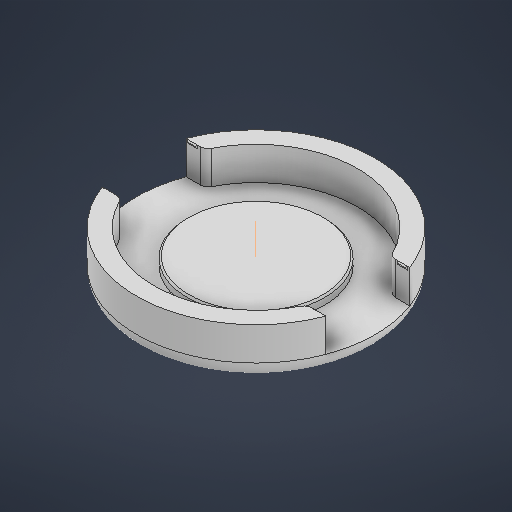
# Autodesk Inventor part: Head Plate Cover Cap
Saved by Autodesk Inventor 2026.1 (Build 301233000, 233)
## iProperties
Created: 2025-10-23
Part Number: Head Plate Cover Cap
Material: Generic
Document SubType Name: Modeling
Designer: mumin
Density: 1 g/cm^3
Appearance: Default
Author: mumin
Autodesk Inventor part; units mm, degrees
ref_plane "YZ Plane" through (0, 0, 0) normal (1, 0, 0) x (0, 1, 0)
ref_plane "XZ Plane" through (0, 0, 0) normal (0, 1, 0) x (-1, 0, 0)
ref_plane "XY Plane" through (0, 0, 0) normal (0, 0, 1) x (1, 0, 0)
sketch "Sketch1" plane through (0, 0, 0) normal (0, 1, 0) x (-1, 0, 0)
  circle A0 centre (0, 0) radius 42.1
  arc A1 (54.3341, 27.7273) -> (-54.3341, 27.7273) centre (0, 0) ccw
  line L0 (0, 0) -> (0, -61)
  line L1 (0, 0) -> (0, 0)
  line L2 (-117.5, 20) -> (-117.5, -20)
  line L3 (117.5, -20) -> (117.5, 20)
  line L4 (117.5, 25) -> (-117.5, -25) construction
  line L5 (-117.5, 25) -> (117.5, -25) construction
  line L6 (112.5, 25) -> (58.7878, 25)
  line L7 (-58.7878, 25) -> (-112.5, 25)
  line L8 (58.7878, -25) -> (112.5, -25)
  line L9 (-112.5, -25) -> (-58.7878, -25)
  arc A2 (-54.3341, -27.7273) -> (54.3341, -27.7273) centre (0, 0) ccw
  arc A3 (112.5, -25) -> (117.5, -20) centre (112.5, -20) ccw
  arc A4 (117.5, 20) -> (112.5, 25) centre (112.5, 20) ccw
  arc A5 (58.7878, -25) -> (54.3341, -27.7273) centre (58.7878, -30) ccw
  arc A6 (54.3341, 27.7273) -> (58.7878, 25) centre (58.7878, 30) ccw
  arc A7 (-54.3341, -27.7273) -> (-58.7878, -25) centre (-58.7878, -30) ccw
  arc A8 (-58.7878, 25) -> (-54.3341, 27.7273) centre (-58.7878, 30) ccw
  arc A9 (-117.5, -20) -> (-112.5, -25) centre (-112.5, -20) ccw
  arc A10 (-112.5, 25) -> (-117.5, 20) centre (-112.5, 20) ccw
  circle A11 centre (0, 0) radius 41.4
  circle A12 centre (0, 0) radius 67
  arc A13 (58.7878, -25.6) -> (54.8686, -28) centre (58.7878, -30) ccw
  line L10 (58.7878, -25.6) -> (112.5, -25.6)
  arc A14 (112.5, -25.6) -> (118.1, -20) centre (112.5, -20) ccw
  line L11 (118.1, -20) -> (118.1, 20)
  arc A15 (118.1, 20) -> (112.5, 25.6) centre (112.5, 20) ccw
  line L12 (112.5, 25.6) -> (58.7878, 25.6)
  arc A16 (54.8686, 28) -> (58.7878, 25.6) centre (58.7878, 30) ccw
  arc A17 (54.8686, 28) -> (-54.8686, 28) centre (0, 0) ccw
  arc A18 (-58.7878, 25.6) -> (-54.8686, 28) centre (-58.7878, 30) ccw
  line L13 (-58.7878, 25.6) -> (-112.5, 25.6)
  arc A19 (-112.5, 25.6) -> (-118.1, 20) centre (-112.5, 20) ccw
  line L14 (-118.1, 20) -> (-118.1, -20)
  arc A20 (-118.1, -20) -> (-112.5, -25.6) centre (-112.5, -20) ccw
  line L15 (-112.5, -25.6) -> (-58.7878, -25.6)
  arc A21 (-54.8686, -28) -> (-58.7878, -25.6) centre (-58.7878, -30) ccw
  arc A22 (-54.8686, -28) -> (54.8686, -28) centre (0, 0) ccw
  circle A23 centre (0, 0) radius 72
  line L16 (-112.5, 25.3) -> (-58.7878, 25.3)
  arc A24 (-58.7878, 25.3) -> (-54.6014, 27.8636) centre (-58.7878, 30) ccw
  arc A25 (54.6014, 27.8636) -> (-54.6014, 27.8636) centre (0, 0) ccw
  arc A26 (54.6014, 27.8636) -> (58.7878, 25.3) centre (58.7878, 30) ccw
  line L17 (58.7878, 25.3) -> (112.5, 25.3)
  arc A27 (117.8, 20) -> (112.5, 25.3) centre (112.5, 20) ccw
  line L18 (117.8, 20) -> (117.8, -20)
  arc A28 (112.5, -25.3) -> (117.8, -20) centre (112.5, -20) ccw
  line L19 (112.5, -25.3) -> (58.7878, -25.3)
  arc A29 (58.7878, -25.3) -> (54.6014, -27.8636) centre (58.7878, -30) ccw
  arc A30 (-54.6014, -27.8636) -> (54.6014, -27.8636) centre (0, 0) ccw
  arc A31 (-54.6014, -27.8636) -> (-58.7878, -25.3) centre (-58.7878, -30) ccw
  line L20 (-58.7878, -25.3) -> (-112.5, -25.3)
  arc A32 (-117.8, -20) -> (-112.5, -25.3) centre (-112.5, -20) ccw
  line L21 (-117.8, -20) -> (-117.8, 20)
  arc A33 (-112.5, 25.3) -> (-117.8, 20) centre (-112.5, 20) ccw
  point P0 (0, 0)
  point P1 (0, -61)
  point P2 (55.6417, -25)
  point P3 (55.6417, 25)
  point P4 (-55.6417, 25)
  point P5 (-55.6417, -25)
  point P6 (61.9164, 25.6)
  point P7 (-61.9164, 25.6)
  point P8 (-61.9164, -25.6)
  point P9 (61.9164, -25.6)
  point P10 (-67.2952, -25.6)
  point P11 (67.2952, -25.6)
  point P12 (67.2952, 25.6)
  point P13 (-67.2952, 25.6)
  point P14 (-67.4085, -25.3)
  point P15 (67.4085, -25.3)
  point P16 (-67.4085, 25.3)
  point P17 (67.4085, 25.3)
  dimension "d0" = 84.2
  dimension "d1" = 61
  dimension "d2" = 235
  dimension "d3" = 50
  dimension "d4" = 5
  dimension "d5" = 0.7
  dimension "d6" = 134
  dimension "d7" = 0.6
  dimension "d19" = 5
  dimension "d21" = 0.3
  constraints: 64 point on circle, 44 end point, 34 centre point, 16 tangent, 15 parallel, 12 point on line, 7 equal radius, 6 perpendicular, 5 coincident, 3 horizontal, 2 midpoint, 1 vertical, 1 vertical alignment, 30 other
  measures "d0" diameter of A0
  measures "d1" radius of A1
  measures "d2" distance of L5.end L4.end
  measures "d3" distance of L4.end L5.start
  measures "d4" radius of A3
  measures "d5" radial gap between concentric circles of A0 A11
  measures "d6" diameter of A12
  measures "d7" radial gap between concentric circles of A2 A22
  measures "d19" radial gap between concentric circles of A12 A23
  measures "d21" distance between parallel lines of L13 L16
extrude "Friction Fit Shapes" add sketch "Sketch1" along normal blind 5 contours A11
sketch "Sketch2" plane through (0, 0, 0) normal (0, -1, 0) x (1, 0, 0)
  circle A0 centre (0, 0) radius 67
  circle A1 centre (0, 0) radius 72
  dimension "d20" = 5
  constraints: 2 centre point, 1 coincident
  measures "d20" radial gap between concentric circles of A0 A1
extrude "Cap" add sketch "Sketch2" along normal blind 10 contours A0 | A1
fillet "Cap Fillet" radius 10 1 edges at (-72, -10, 0)
extrude "Extrusion3" add sketch "Sketch1" along normal blind 20 contours L17 A26 A25 A24 L16 A12 L13 A18 A17 A16 L12 | A12 L12 A23 L17 | L16 A23 L13 A12 | L12 A16 A17 A18 L13 A12 | A12 L13 A23 L12 | L20 A31 A30 A29 L19 A12 L10 A13 A22 A21 L15 | A12 L15 A23 L20 | L19 A23 L10 A12 | L15 A21 A22 A13 L10 A12 | A12 L10 A23 L15
fillet "Bottom Edge Fillet" [suppressed]
chamfer "Inside edge chamfer" distance 1 angle 45 1 edges at (41.4, 5, 0)
sketch "Sketch3" plane through (67.4085, 0, 25.3) normal (0, 0, -1) x (-1, 0, 0)
  line L0 (0, 20) -> (8.6208, 20) projected
  line L1 (1.3103, 20) -> (7.3103, 20)
  line L2 (7.3103, 20) -> (7.3103, 18)
  line L3 (7.3103, 18) -> (1.3103, 18)
  line L4 (1.3103, 18) -> (1.3103, 20)
  line L5 (8.6208, 0) -> (8.6208, 20) projected
  line L6 (0, 0) -> (0, 20) projected
  point P0 (67.4085, 0)
  point P1 (7.3103, 20)
  dimension "d22" = 6
  dimension "d23" = 2
  dimension "d24" = 1.3105
  dimension "d25" = 1.3103
  constraints: 8 end point, 2 parallel, 1 horizontal, 1 perpendicular, 1 point on line
  measures "d22" distance between parallel lines of L2 L4
  measures "d23" distance between parallel lines of L3 L0
  measures "d24" distance between parallel lines of L5 L2
  measures "d25" distance between parallel lines of L6 L4
extrude "Extrusion4" add sketch "Sketch3" along normal blind 2 draft -45
fillet "Fillet3" radius 0.4 1 edges at (63.0983, 19, 24.3)
ref_plane "Work Plane1" through (0, 0, 0) normal (0, 0, -1) x (0, 1, 0)
pattern_linear "Rectangular Pattern1" count 2 spacing 126.5 along (-1, 0, 0) of "Extrusion4", "Fillet3"
mirror "Mirror1" about plane through (0, 0, 0) normal (0, 0, -1) of "Extrusion4", "Fillet3", "Rectangular Pattern1"
body "Solid1"
